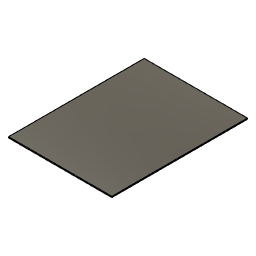
laminaExtractor (Autodesk Fusion 360 design; units mm, degrees)
Autodesk Fusion 360 part; units mm, degrees
sketch "Boceto1" plane through (0, 0, 0) normal (0, 0, 1) x (1, 0, 0)
  line L0 (-100.2237, 25.1698) -> (-1.2237, 25.1698)
  line L1 (-1.2237, 25.1698) -> (-1.2237, -104.8302)
  line L2 (-1.2237, -104.8302) -> (-100.2237, -104.8302)
  line L3 (-100.2237, -104.8302) -> (-100.2237, 25.1698)
  dimension "d1" = 99
  dimension "d2" = 130
  constraint horizontal L0
  constraint vertical L1
  constraint horizontal L2
  constraint vertical L3
  measures "d1" distance of L0.start L0.end
  measures "d2" distance of L0.start L2.end
extrude "Extruir1" add sketch "Boceto1" along normal blind 1
